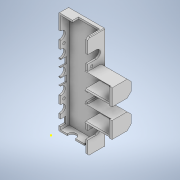
# Autodesk Inventor part: Part1
Saved by Autodesk Inventor 2022 (Build 260153000, 153)
## iProperties
Created: 2020-04-25
Part Number: Part1
Material: Generic
Document SubType Name: Modeling
Designer: Martijn
Density: 1 g/cm^3
Appearance: Default
Author: Martijn
Autodesk Inventor part; units mm, degrees
ref_plane "YZ Plane" through (0, 0, 0) normal (1, 0, 0) x (0, 1, 0)
ref_plane "XZ Plane" through (0, 0, 0) normal (0, 1, 0) x (-1, 0, 0)
ref_plane "XY Plane" through (0, 0, 0) normal (0, 0, 1) x (1, 0, 0)
sketch "Sketch1" plane through (0, 0, 0) normal (0, 0, 1) x (1, 0, 0)
  line L0 (0, 0) -> (0, 156)
  line L1 (0, 156) -> (56, 156)
  line L2 (56, 156) -> (56, 112)
  line L3 (56, 112) -> (96, 112)
  line L4 (96, 112) -> (96, 87)
  line L5 (96, 87) -> (56, 87)
  line L6 (56, 87) -> (56, 69)
  line L7 (56, 69) -> (96, 69)
  line L8 (96, 69) -> (96, 44)
  line L9 (96, 44) -> (56, 44)
  line L10 (56, 44) -> (56, 0)
  line L11 (56, 0) -> (0, 0)
  dimension "d0" = 156
  dimension "d1" = 56
  dimension "d2" = 44
  dimension "d3" = 44
  dimension "d4" = 25
  dimension "d5" = 25
  dimension "d6" = 40
  constraints: 24 end point, 8 perpendicular, 5 point on line, 2 vertical
  measures "d0" distance of L0.start L0.end
  measures "d1" distance of L0.end L1.end
  measures "d2" distance of L1.end L2.end
  measures "d3" distance of L9.end L10.end
  measures "d4" distance between parallel lines of L5 L3
  measures "d5" distance between parallel lines of L9 L7
  measures "d6" distance between parallel lines of L2 L4
extrude "Extrusion1" add sketch "Sketch1" along normal blind 1
sketch "Sketch2" plane through (0, 0, 1) normal (0, 0, 1) x (1, 0, 0)
  line L0 (2.8, 153.2) -> (2.8, 2.8)
  line L1 (2.8, 2.8) -> (53.2, 2.8)
  line L2 (53.2, 2.8) -> (53.2, 45.5)
  line L3 (53.2, 45.5) -> (94.5, 45.5)
  line L4 (94.5, 45.5) -> (94.5, 67.5)
  line L5 (94.5, 67.5) -> (53.2, 67.5)
  line L6 (53.2, 67.5) -> (53.2, 88.5)
  line L7 (53.2, 88.5) -> (94.5, 88.5)
  line L8 (94.5, 88.5) -> (94.5, 110.5)
  line L9 (94.5, 110.5) -> (53.2, 110.5)
  line L10 (53.2, 110.5) -> (53.2, 153.2)
  line L11 (53.2, 153.2) -> (2.8, 153.2)
  line L12 (56, 156) -> (0, 156) projected
  line L13 (0, 156) -> (0, 0) projected
  line L14 (0, 0) -> (56, 0) projected
  line L15 (56, 0) -> (56, 44) projected
  line L16 (96, 69) -> (56, 69) projected
  line L17 (56, 44) -> (96, 44) projected
  line L18 (96, 44) -> (96, 69) projected
  line L19 (96, 112) -> (56, 112) projected
  line L20 (56, 87) -> (96, 87) projected
  line L21 (56, 112) -> (56, 156) projected
  line L22 (0, 156) -> (56, 156)
  line L23 (56, 156) -> (56, 112)
  line L24 (56, 112) -> (96, 112)
  line L25 (96, 87) -> (96, 112) projected
  line L26 (96, 87) -> (56, 87)
  line L27 (56, 69) -> (56, 87) projected
  line L28 (56, 69) -> (96, 69)
  line L29 (96, 44) -> (96, 69) projected
  line L30 (96, 44) -> (56, 44)
  line L31 (56, 0) -> (0, 0)
  line L32 (0, 156) -> (0, 0)
  line L33 (56, 87) -> (56, 69)
  line L34 (96, 112) -> (96, 87)
  line L35 (96, 69) -> (96, 44)
  line L36 (56, 44) -> (56, 0)
  dimension "d9" = 2.8
  dimension "d10" = 2.8
  dimension "d11" = 2.8
  dimension "d12" = 2.8
  dimension "d13" = 1.5
  dimension "d14" = 1.5
  dimension "d15" = 1.5
  dimension "d16" = 1.5
  dimension "d17" = 1.5
  constraints: 48 end point, 10 perpendicular, 5 collinear, 5 point on line, 3 parallel, 2 horizontal, 2 vertical
  measures "d9" distance between parallel lines of L11 L12
  measures "d10" distance between parallel lines of L13 L0
  measures "d11" distance between parallel lines of L14 L1
  measures "d12" distance between parallel lines of L15 L2
  measures "d13" distance between parallel lines of L16 L5
  measures "d14" distance between parallel lines of L17 L3
  measures "d15" distance between parallel lines of L18 L4
  measures "d16" distance between parallel lines of L19 L9
  measures "d17" distance between parallel lines of L20 L7
extrude "Extrusion2" add sketch "Sketch2" along normal blind 25
sketch "Sketch3" plane through (0, 0, 1) normal (0, 0, 1) x (1, 0, 0)
  line L0 (53.2, 67.5) -> (53.2, 88.5) projected
  line L1 (94.5, 110.5) -> (53.2, 110.5)
  line L2 (53.2, 110.5) -> (53.2, 88.5)
  line L3 (53.2, 88.5) -> (94.5, 88.5)
  line L4 (94.5, 88.5) -> (94.5, 110.5)
  line L5 (94.5, 67.5) -> (53.2, 67.5) projected
  line L6 (53.2, 2.8) -> (53.2, 45.5) projected
  line L7 (94.5, 67.5) -> (53.2, 67.5)
  line L8 (53.2, 67.5) -> (53.2, 45.5)
  line L9 (53.2, 45.5) -> (94.5, 45.5)
  line L10 (94.5, 45.5) -> (94.5, 67.5)
  point P0 (0, 0)
  point P1 (53.2, 67.5)
  constraints: 16 end point, 4 parallel, 2 horizontal, 2 perpendicular
extrude "Extrusion3" add sketch "Sketch3" along normal blind 4
sketch "Sketch4" plane through (0, 0, 0) normal (-1, 0, 0) x (0, 0, 1)
  arc A0 (13, 132.8) -> (13, 120.2) centre (13, 126.5) ccw
  line L0 (13, 132.8) -> (26, 132.8)
  line L1 (26, 132.8) -> (26, 120.2)
  line L2 (26, 156) -> (26, 0) projected
  line L3 (13, 120.2) -> (26, 120.2)
  line L4 (1, 2.8) -> (1, 153.2) projected
  line L5 (13, 120.2) -> (13, 132.8)
  line L6 (0, 112) -> (0, 156) projected
  point P0 (0, 0)
  point P1 (26, 153.2)
  dimension "d22" = 6.3
  dimension "d23" = 12
  dimension "d24" = 26.7
  constraints: 8 end point, 3 point on circle, 1 centre point, 1 collinear, 1 horizontal, 1 midpoint, 1 parallel, 1 perpendicular, 1 point on line, 1 tangent
  measures "d22" radius of A0
  measures "d23" distance from line of L4 A0.centre
  measures "d24" vertical distance of point (26, 153.2) A0.centre
extrude "Extrusion4" cut sketch "Sketch4" against normal blind 10
pattern_linear "Rectangular Pattern1" count 5 spacing 24.25 along (0, -1, 0) of "Extrusion4"
sketch "Sketch6" plane through (56, 0, 0) normal (1, 0, 0) x (0, 0, -1)
  line L0 (-26, 0) -> (-26, 44) projected
  line L1 (-26, 21.7) -> (-26, 34.3)
  line L2 (-26, 34.3) -> (-13, 34.3)
  arc A0 (-13, 21.7) -> (-13, 34.3) centre (-13, 28) ccw
  line L3 (-26, 21.7) -> (-13, 21.7)
  line L4 (-1, 2.8) -> (-1, 153.2) projected
  point P0 (0, 0)
  point P1 (-26, 2.8)
  dimension "d30" = 6.3
  dimension "d31" = 12
  dimension "d32" = 25.2
  constraints: 6 end point, 2 point on circle, 2 point on line, 2 tangent, 1 centre point, 1 horizontal, 1 perpendicular
  measures "d30" radius of A0
  measures "d31" distance from line of L4 A0.centre
  measures "d32" vertical distance of point (-26, 2.8) A0.centre
extrude "Extrusion5" cut sketch "Sketch6" against normal blind 10
pattern_linear "Rectangular Pattern2" count 3 spacing 50 along (0, 1, 0) of "Extrusion5"
sketch "Sketch7" plane through (0, 0, 0) normal (0, -1, 0) x (1, 0, 0)
  line L0 (0, 26) -> (56, 26) projected
  line L1 (38.9, 26) -> (51.5, 26)
  line L2 (51.5, 26) -> (51.5, 13)
  arc A0 (38.9, 13) -> (51.5, 13) centre (45.2, 13) ccw
  line L3 (38.9, 26) -> (38.9, 13)
  line L4 (2.8, 1) -> (53.2, 1) projected
  point P0 (0, 0)
  point P1 (53.2, 26)
  dimension "d38" = 6.3
  dimension "d39" = 12
  dimension "d40" = 8
  constraints: 6 end point, 2 point on circle, 2 point on line, 2 tangent, 2 vertical, 1 centre point
  measures "d38" radius of A0
  measures "d39" distance from line of L4 A0.centre
  measures "d40" horizontal distance of point (53.2, 26) A0.centre
extrude "Extrusion6" cut sketch "Sketch7" against normal blind 10
pattern_linear "Rectangular Pattern3" count 2 spacing 26 along (-1, 0, 0) of "Extrusion6"
sketch "Sketch8" plane through (0, 156, 0) normal (0, 1, 0) x (1, 0, 0)
  line L0 (56, -26) -> (0, -26) projected
  line L1 (46.2, -26) -> (46.2, -9.5)
  line L2 (46.2, -26) -> (28.2, -26)
  line L3 (28.2, -26) -> (28.2, -9.5)
  arc A0 (46.2, -9.5) -> (43.7, -7) centre (43.7, -9.5) ccw
  line L4 (43.7, -7) -> (30.7, -7)
  arc A1 (30.7, -7) -> (28.2, -9.5) centre (30.7, -9.5) ccw
  line L5 (56, 0) -> (0, 0) projected
  point P0 (53.2, -26)
  dimension "d46" = 7
  dimension "d47" = 7
  dimension "d48" = 18
  dimension "d49" = 2.5
  dimension "d50" = 2.5
  constraints: 8 end point, 4 point on circle, 4 tangent, 2 centre point, 2 point on line, 2 vertical, 1 horizontal
  measures "d46" distance between parallel lines of L5 L4
  measures "d47" distance from line of point (53.2, -26) L1
  measures "d48" distance between parallel lines of L1 L3
  measures "d49" radius of A0
  measures "d50" radius of A1
extrude "Extrusion7" cut sketch "Sketch8" against normal blind 10
sketch "Sketch9" plane through (0, 0, 0) normal (-1, 0, 0) x (0, 0, 1)
  line L0 (1, 153.2) -> (1, 2.8) projected
  line L1 (5, 94.875) -> (5, 85.375)
  line L2 (26, 85.375) -> (5, 85.375)
  line L3 (5, 94.875) -> (26, 94.875)
  line L4 (0, 156) -> (26, 156) projected
  line L5 (26, 94.875) -> (26, 85.375)
  line L6 (26, 95.95) -> (26, 84.3) projected
  line L7 (13, 84.3) -> (26, 84.3) projected
  line L8 (26, 95.95) -> (13, 95.95) projected
  point P0 (0, 0)
  point P1 (26, 153.2)
  point P2 (5, 90.125)
  dimension "d56" = 9.5
  dimension "d112" = 4
  dimension "d144" = 11.65
  dimension "d145" = 5.825
  constraints: 8 end point, 2 collinear, 1 horizontal, 1 midpoint, 1 perpendicular
  measures "d56" distance between parallel lines of L3 L2
  measures "d112" distance between parallel lines of L0 L1
  measures "d144" distance between parallel lines of L7 L8
  measures "d145" distance from line of L8 point (5, 90.125)
extrude "Extrusion8" cut sketch "Sketch9" against normal blind 10
pattern_linear "Rectangular Pattern4" count 2 spacing 24.25 along (0, -1, 0) of "Extrusion8"
sketch "Sketch10" plane through (0, 0, 0) normal (-1, 0, 0) x (0, 0, 1)
  line L0 (26, 23.2) -> (26, 0) projected
  line L1 (26, 16.8) -> (6, 16.8)
  line L2 (6, 16.8) -> (6, 6.8)
  line L3 (6, 6.8) -> (26, 6.8)
  line L4 (26, 6.8) -> (26, 16.8)
  line L5 (1, 153.2) -> (1, 2.8) projected
  point P0 (0, 0)
  point P1 (26, 2.8)
  point P2 (3, 64)
  point P3 (1, 2.8)
  point P4 (26, 6.8)
  dimension "d64" = 4
  dimension "d65" = 10
  dimension "d66" = 5
  constraints: 8 end point, 2 parallel, 1 horizontal, 1 perpendicular, 1 point on line, 1 other
  measures "d64" distance from line of point (26, 2.8) L3
  measures "d65" distance between parallel lines of L1 L3
extrude "Extrusion9" cut sketch "Sketch10" against normal blind 10
sketch "Sketch11" plane through (0, 0, 0) normal (-1, 0, 0) x (0, 0, 1)
  line L0 (26, 156) -> (26, 132.8) projected
  line L1 (26, 153) -> (23, 156)
  line L2 (0, 156) -> (26, 156) projected
  line L3 (26, 156) -> (26, 153)
  line L4 (23, 156) -> (26, 156)
  point P0 (0, 0)
  dimension "d69" = 45
  dimension "d70" = 3
  constraints: 6 end point, 2 point on line, 1 perpendicular, 1 vertical
  measures "d69" angle of L0 L1
  measures "d70" distance of L0.start L1.start
extrude "Extrusion10" cut sketch "Sketch11" against normal blind 60
sketch "Sketch12" plane through (0, 0, 0) normal (-1, 0, 0) x (0, 0, 1)
  line L0 (0, 0) -> (26, 0) projected
  line L1 (26, 0) -> (23, 0)
  line L2 (23, 0) -> (26, 3)
  line L3 (26, 21.7) -> (26, 2.8) projected
  line L4 (26, 0) -> (26, 2.8) projected
  line L5 (26, 0) -> (26, 3)
  dimension "d73" = 45
  dimension "d74" = 3
  constraints: 6 end point, 2 point on line, 1 collinear
  measures "d73" angle of L0 L2
  measures "d74" distance from line of L2.end L0
extrude "Extrusion11" cut sketch "Sketch12" against normal blind 60
chamfer "Chamfer1" distance 6 angle 45 4 edges at (76, 112, 0) (76, 87, 0) (76, 69, 0) (76, 44, 0)
sketch "Sketch15" plane through (96, 112, 26) normal (0, 1, 0) x (1, 0, 0)
  line L0 (0, 0) -> (0, -3)
  line L1 (0, -3) -> (-4.5, -3)
  line L2 (-1.5, 21) -> (-1.5, 0) projected
  line L3 (-4.5, -3) -> (-1.5, 0)
  line L4 (-1.5, 0) -> (0, 0)
  line L5 (0, 20) -> (0, 0) projected
  point P0 (-96, 26)
  point P1 (-1.5, 20.5)
  dimension "d86" = 3
  dimension "d87" = 135
  constraints: 8 end point, 1 collinear, 1 parallel, 1 perpendicular, 1 vertical
  measures "d86" distance of L0.start L0.end
  measures "d87" angle of L4 L3
extrude "Extrusion12" add sketch "Sketch15" against normal up to surface (25 mm away)
pattern_linear "Rectangular Pattern5" count 2 spacing 43 along (0, -1, 0) of "Extrusion12"
sketch "Sketch17" plane through (0, 0, 26) normal (0, 0, 1) x (1, 0, 0)
  point P0 (0, 0)
sketch "Sketch18" plane through (0, 0, 26) normal (0, 0, 1) x (1, 0, 0)
  line L0 (2.8, 0) -> (0, 0)
  line L1 (0, 0) -> (0, 156)
  line L2 (0, 156) -> (2.8, 156)
  line L3 (2.8, 156) -> (2.8, 0)
  line L4 (0, 153) -> (0, 132.8) projected
  line L5 (12.9, 0) -> (25.5, 0) projected
  line L6 (0, 156) -> (28.2, 156) projected
  line L7 (2.8, 108.55) -> (2.8, 120.2) projected
  point P0 (0, 0)
  point P1 (2, 0)
  point P2 (2, 156)
  constraints: 8 end point, 4 collinear, 2 parallel, 1 horizontal, 1 perpendicular
extrude "Extrusion13" cut sketch "Sketch18" against normal blind 12
sketch "Sketch19" plane through (53.2, 2.8, 1) normal (-1, 0, 0) x (0, 0, 1)
  line L0 (25, 84.2) -> (25, 85.7)
  line L1 (25, 84.2) -> (26.5, 84.2)
  line L2 (25, 85.7) -> (26.5, 84.2)
  line L3 (25, 107.7) -> (25, 109.2)
  line L4 (25, 118.9) -> (25, 107.7) projected
  line L5 (26.5, 109.2) -> (25, 107.7)
  line L6 (26.5, 109.2) -> (25, 109.2)
  point P0 (-1, -2.8)
  dimension "d100" = 45
  dimension "d105" = 1.5
  dimension "d106" = 1.5
  dimension "d110" = 1.5
  dimension "d111" = 1.5
  constraints: 12 end point, 1 coincident, 1 horizontal, 1 point on line, 1 vertical
  measures "d100" angle of L1 L2
  measures "d105" distance of L0.start L0.end
  measures "d106" distance of L0.start L1.end
  measures "d110" distance of L3.start L3.end
  measures "d111" distance of L5.start L3.end
extrude "Extrusion14" add sketch "Sketch19" against normal up to next
pattern_linear "Rectangular Pattern6" count 2 spacing 43 along (0, -1, 0) of "Extrusion14"
sketch "Sketch20" plane through (2.8, 153.2, 1) normal (0, -1, 0) x (1, 0, 0)
  point P0 (-2.8, -1)
sketch "Sketch21" plane through (2.8, 153.2, 1) normal (0, -1, 0) x (1, 0, 0)
  line L0 (51.1352, 4) -> (18.2, 4)
  line L1 (18.2, 4) -> (18.2, 24.8)
  line L2 (18.2, 24.8) -> (50.4, 24.8)
  line L3 (50.4, 24.8) -> (50.4, 2.2006)
  line L4 (25.4, 24.8) -> (0, 24.8) projected
  line L5 (50.4, 0) -> (50.4, 24.8) projected
  line L6 (50.4, 0) -> (0, 0) projected
  point P0 (-2.8, -1)
  point P1 (50.4, 4)
  dimension "d113" = 32.2
  dimension "d134" = 4
  constraints: 8 end point, 2 collinear, 2 parallel, 1 horizontal, 1 perpendicular
  measures "d113" distance of L1.end L2.end
  measures "d134" distance between parallel lines of L6 L0
extrude "Extrusion15" cut sketch "Sketch21" against normal blind 3
sketch "Sketch22" plane through (0, 126.5, 13) normal (-1, 0, 0) x (0, 0, 1)
  circle A0 centre (-4, -12.125) radius 2
  circle A1 centre (-4, -84.875) radius 2
  line L0 (-4, -12.125) -> (1, -12.125)
  line L1 (1, -17.95) -> (1, -6.3) projected
  line L2 (-12, 26.7) -> (-12, -123.7) projected
  line L3 (-4, -84.875) -> (1, -84.875)
  line L4 (1, -90.7) -> (1, -79.05) projected
  point P0 (-13, -126.5)
  dimension "d116" = 4
  dimension "d117" = 4
  dimension "d119" = 8
  dimension "d120" = 8
  constraints: 4 end point, 2 centre point, 2 midpoint, 2 perpendicular
  measures "d116" diameter of A0
  measures "d117" diameter of A1
  measures "d119" distance from line of L2 L0.start
  measures "d120" distance from line of L2 L3.start
extrude "Extrusion16" cut sketch "Sketch22" against normal blind 10
sketch "Sketch23" plane through (56, 128, 13) normal (1, 0, 0) x (0, 0, -1)
  circle A0 centre (-7, -12) radius 2
  circle A1 centre (-7, -88) radius 2
  line L0 (12, -125.2) -> (12, 25.2) projected
  line L1 (13, 28) -> (-10, 28) projected
  line L2 (13, -128) -> (-10, -128) projected
  dimension "d123" = 4
  dimension "d129" = 4
  dimension "d136" = 19
  dimension "d137" = 19
  dimension "d146" = 40
  dimension "d147" = 40
  constraints: 2 centre point
  measures "d123" diameter of A1
  measures "d129" diameter of A0
  measures "d136" distance from line of L0 A1.centre
  measures "d137" distance from line of L0 A0.centre
  measures "d146" distance from line of L1 A0.centre
  measures "d147" distance from line of L2 A1.centre
extrude "Extrusion17" cut sketch "Sketch23" against normal blind 10
sketch "Sketch24" plane through (2.8, 2.8, 1) normal (0, 1, 0) x (1, 0, 0)
  line L0 (0, 0) -> (50.4, 0) projected
  line L1 (50.4, 0) -> (50.4, -24.8) projected
  line L2 (0, 0) -> (50.4, 0)
  line L3 (50.4, 0) -> (50.4, -24.8)
  line L4 (50.4, -24.8) -> (0, -24.8)
  line L5 (0, -24.8) -> (0, 0)
  point P0 (-2.8, 1)
  constraints: 8 end point, 2 parallel, 1 horizontal, 1 perpendicular
extrude "Extrusion18" cut sketch "Sketch24" against normal blind 0.3
sketch "Sketch25" plane through (53.2, 156, 23) normal (0, 1, 0) x (1, 0, 0)
  line L0 (-32.2, -2.8) -> (-32.2, 0) projected
  line L1 (-50.4, 9) -> (-32.2, 9)
  line L2 (-32.2, 9) -> (-32.2, -2.8)
  line L3 (-32.2, -2.8) -> (-50.4, -2.8)
  line L4 (-50.4, -2.8) -> (-50.4, 9)
  point P0 (-53.2, 23)
  constraints: 8 end point, 2 parallel, 1 horizontal, 1 perpendicular
extrude "Extrusion19" cut sketch "Sketch25" against normal blind 10
sketch "Sketch26" plane through (45.2, 0, 13) normal (0, -1, 0) x (1, 0, 0)
  line L0 (8, -12) -> (8, 12.5) projected
  line L1 (-42.4, 1) -> (8, 1)
  line L2 (8, 1) -> (8, 12.5)
  line L3 (8, 12.5) -> (-42.4, 12.5)
  line L4 (-42.4, 12.5) -> (-42.4, 1)
  point P0 (-45.2, -13)
  point P1 (8, 1)
  constraints: 8 end point, 2 parallel, 1 horizontal, 1 perpendicular
extrude "Extrusion20" cut sketch "Sketch26" against normal blind 10
fillet "Fillet2" radius 1 8 edges at (0, 156, 7) (56, 156, 11.5) (0, 0, 7) (56, 0, 11.5) (0, 94.875, 9.5) (0, 85.375, 9.5) (0, 70.625, 9.5) (0, 61.125, 9.5)
body "Solid1"
